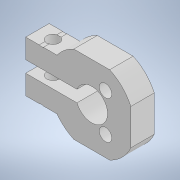
# Autodesk Inventor part: ギア固定具1
Saved by Autodesk Inventor 2021 (Build 250183000, 183)
## iProperties
Created: 2022-02-11
Part Number: ギア固定具1
Material: 一般
Document SubType Name: Modeling
Designer: hirohumi
Density: 1 g/cm^3
Appearance: 既定
Author: hirohumi
Autodesk Inventor part; units mm, degrees
ref_plane "YZ Plane" through (0, 0, 0) normal (1, 0, 0) x (0, 1, 0)
ref_plane "XZ Plane" through (0, 0, 0) normal (0, 1, 0) x (-1, 0, 0)
ref_plane "XY Plane" through (0, 0, 0) normal (0, 0, 1) x (1, 0, 0)
sketch "スケッチ1" plane through (0, 0, 0) normal (0, 0, 1) x (1, 0, 0)
  circle A0 centre (3.5267, 4.8541) radius 1.6
  circle A1 centre (3.5267, -4.8541) radius 1.6
  line L0 (3.5267, 4.8541) -> (0, 0) construction
  line L1 (0, 0) -> (3.5267, -4.8541) construction
  line L2 (0, 0) -> (7.2054, 0) construction
  circle A2 centre (0, 0) radius 4.05
  arc A3 (-8.8741, 6.5) -> (-8.8741, -6.5) centre (0, 0) ccw construction
  line L3 (-8.8741, 6.5) -> (-12.3356, 6.5)
  line L4 (-16.8741, 6.5) -> (-16.8741, 1.5)
  line L5 (-16.8741, 1.5) -> (-3.762, 1.5)
  line L6 (-3.762, -1.5) -> (-16.8741, -1.5)
  line L7 (-16.8741, -1.5) -> (-16.8741, -6.5)
  line L8 (-16.8741, -6.5) -> (-13.4126, -6.5)
  line L9 (-4.5826, 10) -> (4.5826, 10)
  line L10 (-4.5826, -10) -> (4.5826, -10)
  line L11 (10, 4.5826) -> (10, -4.5826)
  circle A4 centre (0, 0) radius 10 construction
  arc A5 (-12.3356, 6.5) -> (-13.4126, 6.5) centre (-12.8741, 7.9) ccw construction
  arc A6 (-12.3356, -6.5) -> (-13.4126, -6.5) centre (-12.8741, -7.9) ccw
  arc A7 (-4.5826, 10) -> (-8.8741, 6.5) centre (0, 0) ccw
  arc A8 (4.5826, 10) -> (-4.5826, 10) centre (0, 0) ccw construction
  arc A9 (10, 4.5826) -> (4.5826, 10) centre (0, 0) ccw
  arc A10 (10, -4.5826) -> (10, 4.5826) centre (0, 0) ccw construction
  arc A11 (4.5826, -10) -> (10, -4.5826) centre (0, 0) ccw
  arc A12 (-4.5826, -10) -> (4.5826, -10) centre (0, 0) ccw construction
  arc A13 (-8.8741, -6.5) -> (-4.5826, -10) centre (0, 0) ccw
  arc A14 (-13.4126, 6.5) -> (-12.3356, 6.5) centre (-12.8741, 7.9) ccw
  line L12 (-13.4126, 6.5) -> (-16.8741, 6.5)
  line L13 (-12.3356, 6.5) -> (-13.4126, 6.5) construction
  arc A15 (-13.4126, -6.5) -> (-12.3356, -6.5) centre (-12.8741, -7.9) ccw construction
  line L14 (-13.4126, -6.5) -> (-12.3356, -6.5) construction
  line L15 (-12.3356, -6.5) -> (-8.8741, -6.5)
  dimension "d0" = 3.2
  dimension "d1" = 3.2
  dimension "d2" = 6
  dimension "d3" = 6
  dimension "d4" = 108
  dimension "d5" = 54
  dimension "d6" = 8.1
  dimension "d7" = 22
  dimension "d8" = 5
  dimension "d9" = 5
  dimension "d10" = 20
  dimension "d11" = 3
  dimension "d12" = 1.5
  dimension "d13" = 8
  dimension "d14" = 3
  dimension "d15" = 3
  dimension "d16" = 1.4
  dimension "d17" = 1.4
  dimension "d18" = 4
  dimension "d19" = 4
  constraints: 41 point on circle, 32 end point, 16 centre point, 7 perpendicular, 5 horizontal, 3 coincident, 3 point on line, 3 tangent, 2 parallel, 1 vertical
  measures "d0" diameter of A0
  measures "d1" diameter of A1
  measures "d2" distance of L0.end L0.start
  measures "d3" distance of L1.end L0.end
  measures "d4" angle of L1 L0
  measures "d5" angle of L2 L0
  measures "d6" diameter of A2
  measures "d7" diameter of A3
  measures "d8" distance between parallel lines of L5 L3
  measures "d9" distance between parallel lines of L8 L6
  measures "d10" diameter of A4
  measures "d11" distance between parallel lines of L6 L5
  measures "d12" distance from line of L0.end L5
  measures "d13" distance of L3.start L4.start
  measures "d14" diameter of A5
  measures "d15" diameter of A6
  measures "d16" distance from line of L3 A5.centre
  measures "d17" distance from line of A6.centre L8
  measures "d18" distance from line of L4 A5.centre
  measures "d19" distance from line of L7 A6.centre
extrude "押し出し1" add sketch "スケッチ1" along normal blind 6 contours A2 L5 L4 L12 A14 L3 A7 L9 A9 L11 A11 L10 A13 L15 A6 L8 L7 L6
sketch "スケッチ2" plane through (-16.8741, 6.5, 0) normal (0, 1, 0) x (1, 0, 0)
  circle A0 centre (4, -3) radius 1.6
  line L0 (4.5385, 0) -> (3.4615, 0) projected
  point P0 (16.8741, 0)
  point P1 (4, 0)
  dimension "d22" = 3.2
  dimension "d23" = 3
  constraints: 1 centre point, 1 midpoint, 1 vertical alignment
  measures "d22" diameter of A0
  measures "d23" distance of point (4, 0) A0.centre
extrude "押し出し2" cut sketch "スケッチ2" against normal through all
equation "\"d5\" = 0.5 * d4"
equation "\"d12\" = 0.5 * d11"
